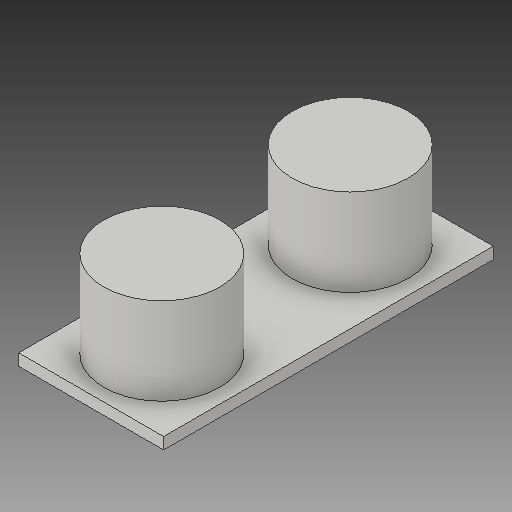
# Autodesk Inventor part: Sonar
Saved by Autodesk Inventor 2018 (Build 220112000, 112)
## iProperties
Created: 2017-10-07
Part Number: Sonar
Material: Generic
Document SubType Name: Modeling
Designer: Akram Al-Hourani
Density: 1 g/cm^3
Appearance: Default
Mass: 6.28149 g
Surface Area: 32.3597 cm^2
Volume: 6.28149 cm^3
Author: Akram Al-Hourani
Autodesk Inventor part; units mm, degrees
ref_plane "YZ Plane" through (0, 0, 0) normal (1, 0, 0) x (0, 1, 0)
ref_plane "XZ Plane" through (0, 0, 0) normal (0, 1, 0) x (-1, 0, 0)
ref_plane "XY Plane" through (0, 0, 0) normal (0, 0, 1) x (1, 0, 0)
sketch "Sketch1" plane through (0, 0, 0) normal (0, 1, 0) x (-1, 0, 0)
  line L0 (-10, 22.75) -> (10, 22.75)
  line L1 (10, 22.75) -> (10, -22.75)
  line L2 (10, -22.75) -> (-10, -22.75)
  line L3 (-10, -22.75) -> (-10, 22.75)
  line L4 (-10, 22.75) -> (10, -22.75) construction
  line L5 (10, 22.75) -> (-10, -22.75) construction
  point P0 (0, 0)
  dimension "d0" = 20
  dimension "d1" = 45.5
  constraints: 12 end point, 2 midpoint, 2 parallel, 1 horizontal, 1 perpendicular
  measures "d0" distance of L1.end L2.end
  measures "d1" distance of L0.end L1.end
extrude "Extrusion1" add sketch "Sketch1" along normal blind 1.6
sketch "Sketch2" plane through (0, 1.6, 0) normal (0, 1, 0) x (1, 0, 0)
  line L0 (0, 0) -> (0, 21) construction
  line L1 (0, 21) -> (0, 13) construction
  circle A0 centre (0, 13) radius 8
  line L2 (0, 0) -> (0, -13) construction
  circle A1 centre (0, -13) radius 8
  dimension "d4" = 21
  dimension "d5" = 8
  dimension "d6" = 16
  dimension "d7" = 13
  dimension "d8" = 16
  constraints: 6 end point, 2 centre point, 2 coincident, 2 vertical, 1 point on line
  measures "d4" distance of L0.start L0.end
  measures "d5" distance of L0.end L1.end
  measures "d6" diameter of A0
  measures "d7" distance of L0.start L2.end
  measures "d8" diameter of A1
extrude "Extrusion2" add sketch "Sketch2" along normal blind 12
body "Solid1"
